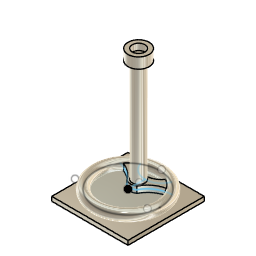
TORP (Autodesk Fusion 360 design; units mm, degrees)
Autodesk Fusion 360 part; units mm, degrees
sketch "Sketch1" plane through (0, 0, 0) normal (0, 0, 1) x (1, 0, 0)
  circle A0 centre (0, 0) radius 0.3
  dimension "d1" = 0.6
  constraint coincident A0.centre origin
  measures "d1" diameter of A0
extrude "Extrude1" add sketch "Sketch1" along normal blind 5 makes body 1
sketch "Sketch2" plane through (0, 0, 5) normal (0, 0, 1) x (-1, 0, 0)
  circle A0 centre (0, 0) radius 0.3
  circle A1 centre (0, 0) radius 0.5
  dimension "d4" = 1
  constraint coincident A0.centre A1.centre
  measures "d4" diameter of A1
extrude "Extrude2" add sketch "Sketch2" along normal blind 0.5 contours A0 | A1 bodies 1
shell "Shell1" thickness 0.2 removed faces 1 at (-0.3557, 0.1033, 5.5) on bodies 1
torus "TorusPrimitive1" add centre line diameter 3 section diameter 0.5 placed x (1, 0, 0) y (0, 1, 0) z (0, 0, 1) at (0, 0, 0) separate body makes body 2
move_body "Move1" bodies 1 to x (1, 0, 0) y (0, 1, 0) z (0, 0, 1) at (0, 0.5, 0)
sketch "Sketch4" plane through (0, 0, 0) normal (0, 0, 1) x (1, 0, 0)
extrude "Extrude3" add 1 faces at (0.2548, 0.4968, 0) along direction (0, 0, -1) blind 0.25 on bodies 1 bodies 1
sketch "Sketch6" plane through (0, 0, 0) normal (0, 0, 1) x (1, 0, 0)
  circle A0 centre (0, 0) radius 1.5
  arc A1 (-1.11, 1.0089) -> (1.0949, 1.0252) centre (-0.01, 1.3523) ccw
  arc A2 (-0.7508, 1.2986) -> (0.7106, 1.321) centre (-0.0242, 1.5781) ccw
  dimension "d14" = 3
  constraint coincident A0.centre origin
  constraint coincident A0 A1.start
  constraint coincident A0 A1.end
  constraint coincident A0 A2.start
  constraint coincident A0 A2.end
  measures "d14" diameter of A0
sketch "Sketch7" plane through (0, 0, 0) normal (1, 0, 0) x (0, 1, 0)
sketch "Sketch8" plane through (0, 0, 0) normal (0, 0, 1) x (1, 0, 0)
  circle A0 centre (0, 0) radius 1.5
  arc A1 (-0.7335, 1.3084) -> (0.7335, 1.3084) centre (0, 1.5833) ccw
  arc A2 (-0.2284, 0.1788) -> (-1.2246, 0.8662) centre (-1.6631, -0.8348) ccw
  line L0 (0, 0.8) -> (0, 0.19)
  line L1 (0, 0.8) -> (0, 0.19)
  arc A3 (1.2625, 0.81) -> (0.2355, 0.1827) centre (1.2653, -0.3489) ccw
  arc A4 (-0.2284, 0.1788) -> (0.2355, 0.1827) centre (0.0007, 0.5253) ccw
  dimension "d21" = 3
  constraint coincident A0.centre origin
  constraint coincident A0 A1.start
  constraint coincident A0 A1.end
  constraint coincident A0 A2.end
  constraint midpoint A1 L0.start
  constraint vertical L0
  constraint coincident A0 A3.start
  measures "d21" diameter of A0
extrude "Extrude9" add sketch "Sketch8" along normal mid plane 0.3 contours A0 A1 A2 A3 A4 bodies 1 2
extrude "Extrude10" cut 1 faces at (0.2548, 0.4968, -0.25) along direction (0, 0, 1) blind 0.1 on bodies 1 bodies 1
sketch "Sketch11" plane through (0, 0, 0) normal (0, 0, 1) x (1, 0, 0)
  line L0 (-1.8, 1.8) -> (1.8, 1.8)
  line L1 (1.8, 1.8) -> (1.8, -1.8)
  line L2 (1.8, -1.8) -> (-1.8, -1.8)
  line L3 (-1.8, -1.8) -> (-1.8, 1.8)
  line L4 (-1.8, 1.8) -> (1.8, -1.8) construction
  line L5 (1.8, 1.8) -> (-1.8, -1.8) construction
  constraint horizontal L0
  constraint perpendicular L0 L1
  constraint parallel L0 L2
  constraint parallel L1 L3
  constraint coincident L4 origin
  constraint coincident L5 origin
extrude "Extrude11" add sketch "Sketch11" along normal blind 0.2 from surface at -0.5 separate body makes body 3
